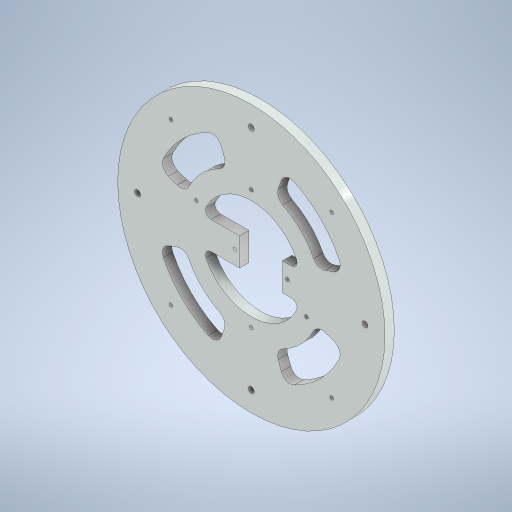
# Autodesk Inventor part: 아크릴 빛번짐
Saved by Autodesk Inventor 2023 (Build 270158000, 158)
## iProperties
Created: 2022-06-05
Part Number: 아크릴 빛번짐
Material: 일반
Document SubType Name: Modeling
Designer: fly01
Density: 1 g/cm^3
Appearance: 기본값
Author: fly01
Autodesk Inventor part; units mm, degrees
ref_plane "YZ Plane" through (0, 0, 0) normal (1, 0, 0) x (0, 1, 0)
ref_plane "XZ Plane" through (0, 0, 0) normal (0, 1, 0) x (-1, 0, 0)
ref_plane "XY Plane" through (0, 0, 0) normal (0, 0, 1) x (1, 0, 0)
sketch "스케치1" plane through (0, 0, 0) normal (0, 0, 1) x (1, 0, 0)
  circle A0 centre (0, 0) radius 27
  circle A1 centre (0, 0) radius 71.7255
  dimension "d0" = 54
  dimension "d1" = 143.451
  constraints: 2 centre point, 2 coincident
  measures "d0" diameter of A0
  measures "d1" diameter of A1
extrude "돌출1" add sketch "스케치1" along normal blind 5
sketch "스케치2" plane through (0, 0, 5) normal (0, 0, 1) x (1, 0, 0)
  circle A0 centre (0, 0) radius 32
  circle A1 centre (0, 32) radius 0.95
  circle A2 centre (0, -32) radius 0.95
  line L0 (0, 0) -> (0, -32) construction
  line L1 (0, 0) -> (29.5641, -12.2459) construction
  circle A3 centre (29.5641, -12.2459) radius 0.95
  line L2 (0, 0) -> (-29.5641, 12.2459) construction
  circle A4 centre (-29.5641, 12.2459) radius 0.95
  dimension "d4" = 64
  dimension "d5" = 1.9
  dimension "d6" = 1.9
  dimension "d7" = 1.9
  dimension "d8" = 67.5
  dimension "d9" = 1.9
  constraints: 6 end point, 5 centre point, 5 point on circle, 2 coincident, 1 collinear, 1 vertical
  measures "d4" diameter of A0
  measures "d5" diameter of A1
  measures "d6" diameter of A2
  measures "d7" diameter of A3
  measures "d8" angle of L1 L0
  measures "d9" diameter of A4
extrude "돌출2" cut sketch "스케치2" against normal blind 10 contours A1 A0 | A0 A1 | A3 A0 | A0 A3 | A4 A0 | A0 A4 | A2 A0 | A0 A2
sketch "스케치3" plane through (0, 0, 0) normal (0, 0, -1) x (-1, 0, 0)
  circle A0 centre (0, 0) radius 61
  circle A1 centre (61, 0) radius 1.6
  circle A2 centre (0, 61) radius 1.6
  circle A3 centre (-61, 0) radius 1.6
  circle A4 centre (0, -61) radius 1.6
  dimension "d12" = 122
  dimension "d13" = 3.2
  dimension "d16" = 360
  constraints: 4 centre point, 1 coincident, 1 horizontal alignment, 11 other
  measures "d13" diameter of A1
extrude "돌출3" cut sketch "스케치3" against normal blind 10 contours A0 A1 | A0 A1 | A2 A0 | A0 A2 | A4 A0 | A0 A4 | A3 A0 | A0 A3
sketch "스케치4" plane through (0, 0, 0) normal (0, 0, -1) x (-1, 0, 0)
  circle A0 centre (0, 0) radius 2.5
  line L0 (0, 0) -> (8.85, 0)
  line L1 (0, 0) -> (-19.35, 0)
  circle A1 centre (8.85, 0) radius 0.95
  circle A2 centre (-19.35, 0) radius 0.95
  line L2 (-29.4038, 7.5) -> (29.4038, 7.5)
  line L3 (29.4038, 7.5) -> (29.4038, -7.5)
  line L4 (29.4038, -7.5) -> (-29.4038, -7.5)
  line L5 (-29.4038, -7.5) -> (-29.4038, 7.5)
  line L6 (-29.4038, 7.5) -> (29.4038, -7.5) construction
  line L7 (29.4038, 7.5) -> (-29.4038, -7.5) construction
  line L8 (-5, -7.5) -> (6.3, -7.5)
  line L9 (10.85, 7.5) -> (6.3, 7.5)
  line L10 (6.3, 7.5) -> (6.3, -7.5)
  line L11 (6.3, -7.5) -> (10.85, -7.5)
  line L12 (10.85, -7.5) -> (10.85, 7.5) construction
  line L13 (-16.8, 7.5) -> (-21.35, 7.5)
  line L14 (-21.35, 7.5) -> (-21.35, -7.5) construction
  line L15 (-21.35, -7.5) -> (-16.8, -7.5)
  line L16 (-16.8, -7.5) -> (-16.8, 7.5)
  point P0 (-16.8, -7.5)
  point P1 (6.3, -7.5)
  point P2 (6.3, 7.5)
  dimension "d20" = 5
  dimension "d21" = 8.85
  dimension "d22" = 19.35
  dimension "d23" = 1.9
  dimension "d24" = 1.9
  dimension "d25" = 15
  dimension "d29" = 16.8
  dimension "d30" = 21.35
  dimension "d31" = 10.85
  dimension "d32" = 6.3
  constraints: 34 end point, 6 parallel, 5 horizontal, 4 point on line, 3 centre point, 3 coincident, 3 perpendicular, 2 midpoint
  measures "d20" diameter of A0
  measures "d21" distance of L0.start L0.end
  measures "d22" distance of L0.start L1.end
  measures "d23" diameter of A1
  measures "d24" diameter of A2
  measures "d25" distance of L2.end L3.end
  measures "d29" distance from line of L16 point (0, 0)
  measures "d30" distance from line of L0.start L14
  measures "d31" distance from line of L12 point (0, 0)
  measures "d32" distance from line of point (0, 0) L10
extrude "돌출4" add sketch "스케치4" against normal blind 5 contours L10 L2 L3 L4 | L16 L4 L5 L2
fillet "모깎기1" radius 3 4 edges at (-25.9374, -7.5, 2.5) (-25.9374, 7.5, 2.5) (25.9374, -7.5, 2.5) (25.9374, 7.5, 2.5)
sketch "스케치6" plane through (0, 0, 0) normal (0, 0, -1) x (-1, 0, 0)
  circle A0 centre (0, 0) radius 52.5
  circle A1 centre (0, 0) radius 37.5
  line L0 (0, 0) -> (0, -83.3327)
  line L1 (0, 0) -> (22.8876, -62.8832)
  line L2 (0, 0) -> (58.8648, -21.425)
  point P0 (49.3339, -17.9561)
  point P1 (35.2385, -12.8258)
  point P2 (12.8258, -35.2385)
  point P3 (17.9561, -49.3339)
  dimension "d34" = 105
  dimension "d35" = 75
  dimension "d36" = 20
  dimension "d37" = 50
  constraints: 6 end point, 2 centre point, 2 coincident, 1 vertical
  measures "d34" diameter of A0
  measures "d35" diameter of A1
  measures "d36" angle of L0 L1
  measures "d37" angle of L1 L2
extrude "돌출5" cut sketch "스케치6" against normal blind 5 contours A0 L1 A1 L2
fillet "모깎기2" radius 5 4 edges at (-35.2385, -12.8258, 2.5) (-49.3339, -17.9561, 2.5) (-17.9561, -49.3339, 2.5) (-12.8258, -35.2385, 2.5)
pattern_circular "원형 패턴1" count 4 over 360 about axis through (0, 0, 0) along (0, 0, 1) of "돌출5", "모깎기2"
sketch "스케치7" plane through (0, 0, 0) normal (0, 0, -1) x (-1, 0, 0)
  circle A0 centre (0, -61) radius 1.6 projected
  circle A1 centre (0, 0) radius 61 construction
  circle A2 centre (43.1335, -43.1335) radius 0.95
  line L0 (43.1335, -43.1335) -> (0, 0) construction
  line L1 (0, 0) -> (0, -16.1996)
  circle A3 centre (43.1335, 43.1335) radius 0.95
  circle A4 centre (-43.1335, 43.1335) radius 0.95
  circle A5 centre (-43.1335, -43.1335) radius 0.95
  dimension "d44" = 1.9
  dimension "d45" = 45
  dimension "d48" = 360
  constraints: 5 centre point, 4 end point, 2 point on circle, 1 coincident, 1 vertical, 9 other
  measures "d44" diameter of A2
  measures "d45" angle of L1 L0
extrude "돌출6" cut sketch "스케치7" against normal blind 5 contours A2 | A3 | A4 | A5
